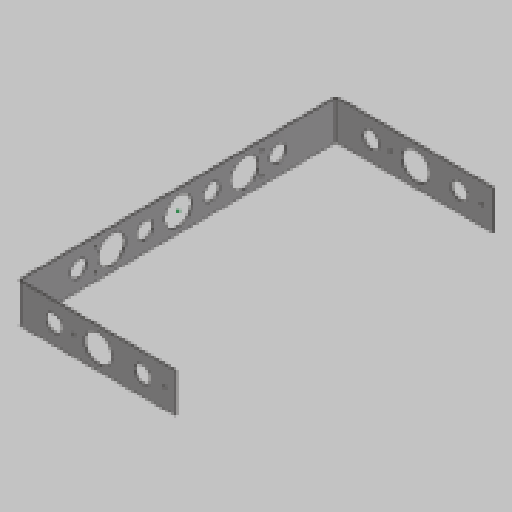
# Autodesk Inventor part: BP-005
Saved by Autodesk Inventor 2023.5 (Build 275446000, 446)
## iProperties
Created: 2025-01-27
Part Number: BP-005
Material: Steel, Alloy
Document SubType Name: Sheet Metal
Designer: slick
Mass: 1993.35 g
Surface Area: 1843.95 cm^2
Volume: 257.871 cm^3
Density: 7.73 g/cm^3
Sheet Metal Rule: Default
Appearance: Semi-Polished
Author: slick
Autodesk Inventor part; units mm, degrees
ref_plane "YZ Plane" through (0, 0, 0) normal (1, 0, 0) x (0, 1, 0)
ref_plane "XZ Plane" through (0, 0, 0) normal (0, 1, 0) x (-1, 0, 0)
ref_plane "XY Plane" through (0, 0, 0) normal (0, 0, 1) x (1, 0, 0)
sketch "Sketch1" plane through (0, 0, 0) normal (1, 0, 0) x (0, 1, 0)
  line L0 (-44.45, -365.125) -> (44.45, -365.125)
  line L1 (44.45, -365.125) -> (44.45, 365.125)
  line L2 (44.45, 365.125) -> (-44.45, 365.125)
  line L3 (-44.45, 365.125) -> (-44.45, -365.125)
  line L4 (-44.45, -365.125) -> (44.45, 365.125) construction
  line L5 (44.45, -365.125) -> (-44.45, 365.125) construction
  point P0 (0, 0)
  dimension "d0" = 88.9
  dimension "d1" = 730.25
  measures "d0" distance of L2.end L1.end
  measures "d1" distance of L1.end L0.end
extrude "Plate1" add sketch "Sketch1" along normal blind 3.048
sketch "Sketch2" plane through (0, -44.45, 362.077) normal (0, 0, 1) x (1, 0, 0)
  line L0 (0, 88.9) -> (0, 0)
  line L1 (0, 0) -> (361.95, 0)
  line L2 (361.95, 0) -> (361.95, 88.9)
  line L3 (361.95, 88.9) -> (0, 88.9)
  constraints: 6 end point, 1 horizontal, 1 perpendicular, 1 vertical
edge flange "Flange1" height 361.95 angle 90 thickness 3.048 bend radius 3.048 thickness toward (0, 0, 1) relief straight relief width 3.048 relief depth 1.524 corner gap 3.048 corner form 0 edges at (3.048, 0, 365.125) (3.048, 0, -365.125) wall of the first edge with corners at (0, 44.45, 362.077) (0, -44.45, 362.077) (361.95, -44.45, 362.077) (361.95, 44.45, 362.077)
bend "Bend1"
corner "Corner1"
sketch "Sketch3" plane through (3.048, 0, 0) normal (1, 0, 0) x (0, 0, -1)
  circle A0 centre (0, 0) radius 31.75
  circle A1 centre (76.2, 0) radius 19.05
  circle A2 centre (152.4, 0) radius 31.75
  circle A3 centre (228.6, 0) radius 19.05
  line L0 (-359.029, 44.45) -> (359.029, 44.45) construction
  line L1 (0, 44.45) -> (0, -44.45) construction
  line L2 (359.029, -44.45) -> (-359.029, -44.45) construction
  circle A4 centre (-76.2, 0) radius 19.05
  circle A5 centre (-152.4, 0) radius 31.75
  circle A6 centre (-228.6, 0) radius 19.05
  dimension "d13" = 63.5
  dimension "d14" = 38.1
  dimension "d15" = 76.2
  dimension "d16" = 76.2
  dimension "d17" = 76.2
  constraints: 7 centre point, 3 horizontal alignment, 3 midpoint, 3 symmetric about line, 2 end point, 2 equal radius, 1 coincident, 3 other
  measures "d13" diameter of A0
  measures "d14" diameter of A1
  measures "d15" distance of A1.centre point (0, 0)
  measures "d16" distance of A2.centre A1.centre
  measures "d17" distance of A2.centre A3.centre
extrude "Cut1" cut sketch "Sketch3" against normal blind 3.048
sketch "Sketch4" plane through (361.95, -44.45, 365.125) normal (0, 0, 1) x (1, 0, 0)
  circle A0 centre (-177.927, 44.45) radius 31.75
  circle A1 centre (-279.527, 44.45) radius 19.05
  circle A2 centre (-76.327, 44.45) radius 19.05
  line L0 (-355.854, 88.9) -> (0, 88.9) projected
  line L1 (0, 88.9) -> (0, 0) projected
  point P0 (-361.95, 44.45)
  point P1 (-177.927, 88.9)
  point P2 (0, 44.45)
  dimension "d21" = 63.5
  dimension "d22" = 38.1
  dimension "d23" = 38.1
  dimension "d24" = 101.6
  dimension "d25" = 101.6
  constraints: 3 centre point, 3 horizontal alignment, 2 midpoint, 1 vertical alignment
  measures "d21" diameter of A0
  measures "d22" diameter of A1
  measures "d23" diameter of A2
  measures "d24" distance of A0.centre A1.centre
  measures "d25" distance of A0.centre A2.centre
extrude "Cut2" cut sketch "Sketch4" against normal up to surface (730.25 mm away)
sketch "Sketch5" plane through (3.048, 0, 0) normal (1, 0, 0) x (0, 0, -1)
  line L0 (-190.5, 25.4) -> (-190.5, -25.4) construction
  line L1 (0, 61.8422) -> (0, -44.45) construction
  line L2 (359.029, -44.45) -> (-359.029, -44.45) projected
  point P0 (0, 0)
  point P1 (-190.5, 0)
  point P2 (190.5, 25.4)
  point P3 (190.5, -25.4)
  dimension "d28" = 50.8
  dimension "d29" = 190.5
  constraints: 4 end point, 2 midpoint, 2 symmetric about line, 2 vertical, 1 horizontal alignment
  measures "d28" distance of L0.start L0.end
  measures "d29" horizontal distance of point (0, 0) L0.start
hole "Hole1" at (3.048, 25.4, 190.5) at (3.048, -25.4, 190.5) at (3.048, 25.4, -190.5) at (3.048, -25.4, -190.5) direction (-1, 0, 0) diameter 6.35 end through all
sketch "Sketch6" plane through (361.95, -44.45, 365.125) normal (0, 0, 1) x (1, 0, 0)
  circle A0 centre (-177.927, 44.45) radius 31.75 projected
  circle A1 centre (-279.527, 44.45) radius 19.05 projected
  circle A2 centre (-76.327, 44.45) radius 19.05 projected
  line L0 (-355.854, 0) -> (-355.854, 88.9) projected
  line L1 (-355.854, 88.9) -> (0, 88.9) projected
  line L2 (0, 88.9) -> (0, 0) projected
  line L3 (0, 0) -> (-355.854, 0) projected
  circle A3 centre (-279.527, 44.45) radius 19.05 projected
  line L4 (-260.477, 44.45) -> (-209.677, 44.45) construction
  point P0 (-361.95, 44.45)
  point P1 (-235.077, 44.45)
  point P2 (-25.527, 44.45)
  point P3 (-235.077, 44.45)
  dimension "d38" = 152.4
  constraints: 5 horizontal alignment, 2 end point, 1 coincident, 1 horizontal, 1 midpoint, 2 other
  measures "d38" distance of point (-25.527, 44.45) point (-177.927, 44.45)
hole "Hole2" at (126.873, 0, 365.125) at (336.423, 0, 365.125) direction (0, 0, -1) diameter 6.35 end through all
sketch "Sketch7" plane through (3.048, 0, 0) normal (1, 0, 0) x (0, 0, -1)
  point P0 (0, 0)
sketch "Sketch8" plane through (3.048, 0, 0) normal (1, 0, 0) x (0, 0, -1)
  circle A0 centre (190.5, 25.4) radius 3.175 projected
  circle A1 centre (-190.5, 25.4) radius 3.175 projected
  circle A2 centre (-190.5, -25.4) radius 3.175 projected
  circle A3 centre (190.5, -25.4) radius 3.175 projected
  circle A4 centre (152.4, 0) radius 31.75 projected
  circle A5 centre (-228.6, 0) radius 19.05 projected
  circle A6 centre (228.6, 0) radius 19.05 projected
  circle A7 centre (76.2, 0) radius 19.05 projected
  circle A8 centre (-76.2, 0) radius 19.05 projected
  circle A9 centre (0, 0) radius 31.75 projected
  circle A10 centre (-152.4, 0) radius 31.75 projected
  line L0 (359.029, -44.45) -> (359.029, 44.45) projected
  line L1 (-359.029, 44.45) -> (359.029, 44.45) projected
  line L2 (-359.029, 44.45) -> (-359.029, -44.45) projected
  line L3 (359.029, -44.45) -> (-359.029, -44.45) projected
  line L4 (-359.029, 44.45) -> (359.029, 44.45) construction
  line L5 (0, 44.45) -> (0, -44.45) construction
  line L6 (359.029, -44.45) -> (-359.029, -44.45) construction
  line L7 (362.077, 44.45) -> (362.077, -44.45) projected
  point P0 (315.3156, 33.3248)
  point P1 (328.0156, 33.3248)
  point P2 (-315.3156, 33.3248)
  point P3 (-328.0156, 33.3248)
  dimension "d47" = 12.7
  dimension "d49" = 11.1252
  dimension "d68" = 34.0614
  constraints: 2 end point, 2 midpoint, 2 symmetric about line, 1 horizontal alignment
  measures "d47" distance of point (328.016, 33.325) point (315.316, 33.325)
  measures "d49" distance from line of L1 point (315.316, 33.325)
  measures "d68" distance from line of L7 point (328.016, 33.325)
hole "Hole3" at (3.048, 33.3248, -315.3156) at (3.048, 33.3248, -328.0156) at (3.048, 33.3248, 328.0156) at (3.048, 33.3248, 315.3156) direction (-1, 0, 0) diameter 5.1054 end through all clearance for "Flat Head Machine Screw (82)" size "#10" standard "Ansi Unified Screw Threads"
sketch "Sketch9" plane through (361.95, -44.45, 365.125) normal (0, 0, 1) x (1, 0, 0)
  circle A0 centre (-235.077, 44.45) radius 3.175 projected
  circle A1 centre (-25.527, 44.45) radius 3.175 projected
  circle A2 centre (-177.927, 44.45) radius 31.75 projected
  circle A3 centre (-279.527, 44.45) radius 19.05 projected
  circle A4 centre (-76.327, 44.45) radius 19.05 projected
  line L0 (-355.854, 88.9) -> (-355.854, 0) projected
  line L1 (0, 0) -> (-355.854, 0) projected
  line L2 (0, 88.9) -> (0, 0) projected
  line L3 (-355.854, 88.9) -> (0, 88.9) projected
  line L4 (-358.902, 88.9) -> (-358.902, 0) projected
  point P0 (-361.95, 44.45)
  point P1 (-324.8406, 77.7748)
  point P2 (-312.1406, 77.7748)
  dimension "d57" = 12.7
  dimension "d59" = 34.0614
  dimension "d60" = 11.1252
  constraints: 1 horizontal alignment
  measures "d57" distance of point (-312.141, 77.775) point (-324.841, 77.775)
  measures "d59" distance from line of point (-324.841, 77.775) L4
  measures "d60" distance from line of L3 point (-324.841, 77.775)
hole "Hole4" at (37.1094, 33.3248, 365.125) at (49.8094, 33.3248, 365.125) direction (0, 0, -1) diameter 5.1054 end through all clearance for "Flat Head Machine Screw (82)" size "#10" standard "Ansi Unified Screw Threads"
equation "\"d19\" = Thickness"
equation "\"d26\" = Thickness"
equation "\"d35\" = Thickness"
equation "\"d55\" = Thickness"
equation "\"d2\" = Thickness"
equation "\"d3\" = BendReliefWidth"
equation "\"d4\" = BendReliefDepth"
equation "\"d5\" = MinimumRemnant"
equation "\"d6\" = TransitionRadius"
equation "\"d9\" = BendRadius"
equation "\"d10\" = CornerReliefSize"
equation "\"d11\" = GapSize"
equation "\"d12\" = JacobiRadiusSize"
equation "\"BendRadius\" = Thickness"
equation "\"BendReliefWidth\" = Thickness"
equation "\"BendReliefDepth\" = 0.5 * Thickness"
equation "\"CornerReliefSize\" = 4 * Thickness"
equation "\"MinimumRemnant\" = 2 * Thickness"
equation "\"TransitionRadius\" = BendRadius"
equation "\"JacobiRadiusSize\" = BendRadius"
equation "\"GapSize\" = Thickness"
equation "\"Thickness\" = 3.048"
body "Solid1"
